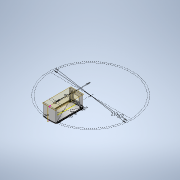
# Autodesk Inventor part: bat_mount001
Saved by Autodesk Inventor 2020 (Build 240168000, 168)
## iProperties
Created: 2024-02-10
Part Number: bat_mount001
Material: Типовые
Document SubType Name: Modeling
Designer: 4s
Density: 1 g/cm^3
Appearance: По умолчанию
Author: 4s
Autodesk Inventor part; units mm, degrees
ref_plane "YZ Plane" through (0, 0, 0) normal (1, 0, 0) x (0, 1, 0)
ref_plane "XZ Plane" through (0, 0, 0) normal (0, 1, 0) x (-1, 0, 0)
ref_plane "XY Plane" through (0, 0, 0) normal (0, 0, 1) x (1, 0, 0)
sketch "Эскиз1" plane through (0, 0, 0) normal (0, 1, 0) x (-1, 0, 0)
  circle A0 centre (0, 0) radius 101 construction
  line L0 (0, 0) -> (0, 101) construction
  line L1 (101, 0) -> (-101, 0) construction
  line L2 (16.8284, 102.0346) -> (-15, 102.0346)
  line L3 (-15, 100.0346) -> (-15, 37.0346)
  line L4 (-13, 37.0346) -> (13, 37.0346)
  line L5 (15, 37.0346) -> (15, 100.0346)
  line L6 (15, 102.0346) -> (-15, 37.0346) construction
  line L7 (-15, 102.0346) -> (15, 37.0346) construction
  arc A1 (15, 100.0346) -> (13, 102.0346) centre (13, 100.0346) ccw
  arc A2 (13, 37.0346) -> (15, 39.0346) centre (13, 39.0346) ccw
  arc A3 (-15, 39.0346) -> (-13, 37.0346) centre (-13, 39.0346) ccw
  arc A4 (-13, 102.0346) -> (-15, 100.0346) centre (-13, 100.0346) ccw
  line L8 (14, 104.0346) -> (-14, 104.0346) construction
  line L9 (-17, 101.0346) -> (-17, 38.0346)
  line L10 (-14, 35.0346) -> (14, 35.0346)
  line L11 (17, 38.0346) -> (17, 101.0346)
  line L12 (17, 104.0346) -> (-17, 35.0346) construction
  line L13 (-17, 104.0346) -> (17, 35.0346) construction
  arc A5 (14, 35.0346) -> (17, 38.0346) centre (14, 38.0346) ccw
  arc A6 (-17, 38.0346) -> (-14, 35.0346) centre (-14, 38.0346) ccw
  arc A7 (-14, 104.0346) -> (-17, 101.0346) centre (-14, 101.0346) ccw
  arc A8 (17, 101.0346) -> (14, 104.0346) centre (14, 101.0346) ccw
  arc A9 (-14.4118, 104.0063) -> (14.4118, 104.0063) centre (0, 0) ccw construction
  arc A10 (14.4118, 104.0063) -> (-14.4118, 104.0063) centre (0, 0) ccw
  line L14 (-15, 102.0346) -> (-16.8284, 102.0346)
  line L15 (-15, 37.0346) -> (-15, 35.2062)
  line L16 (15, 37.0346) -> (15, 35.2062)
  point P0 (0, 69.5346)
  dimension "d2" = 202
  dimension "d3" = 30
  dimension "d4" = 65
  dimension "d5" = 2
  dimension "d6" = 2
  dimension "d7" = 2
  dimension "d8" = 3
  dimension "d9" = 210
  constraints: 34 end point, 29 point on circle, 18 point on line, 17 tangent, 11 centre point, 6 equal radius, 5 midpoint, 4 horizontal, 4 parallel, 3 vertical, 2 coincident, 2 perpendicular, 1 other
  measures "d2" diameter of A0
  measures "d3" distance of L5.start L3.end
  measures "d4" distance of L3.end L2.end
  measures "d5" radius of A1
  measures "d6" distance between parallel lines of L3 L9
  measures "d7" distance between parallel lines of L10 L4
  measures "d8" radius of A5
  measures "d9" diameter of A9
extrude "Выдавливание3" add sketch "Эскиз1" against normal blind 2
ref_plane "РабПлоскость1" through (0, 28, 0) normal (0, 1, 0) x (1, 0, 0)
extrude "Выдавливание1" add sketch "Эскиз1" along normal up to surface (28 mm away) contours L2 L14 A7 A10 A8
ref_plane "РабПлоскость2" through (0, 7, 101.0346) normal (1, 0, 0) x (0, 0, -1)
sketch "Эскиз2" plane through (0, 7, 101.0346) normal (1, 0, 0) x (0, 0, -1)
  line L0 (-1, 0) -> (-1, 21) construction
  line L1 (-1, 21) -> (-2.9716, 21) construction
  line L2 (-2.9716, -9) -> (-2.9716, 21) construction
  line L3 (-2.9716, -9) -> (-2.9716, 21) construction
  line L4 (-2.9716, -9) -> (-2.9716, -9) construction
  line L5 (-2.9716, -9) -> (-2.9716, 21) construction
  line L6 (-2.9716, 21) -> (-2.9716, 21) construction
  line L7 (-2.9716, 21) -> (-2.9716, 21) construction
  line L8 (-1, 21) -> (-2.9716, 21) construction
  line L9 (-2.9716, 21) -> (-1, 21) construction
  line L10 (-1, -7) -> (0, -7) projected
  line L11 (0, -7) -> (63, -7) projected
  line L12 (63, -7) -> (66, -7) projected
  line L13 (66, -7) -> (63, -7) projected
  line L14 (63, -7) -> (0, -7) projected
  line L15 (0, -7) -> (-1, -7) projected
  point P0 (101.0346, -7)
extrude "Выдавливание4" add sketch "Эскиз1" along normal up to surface (28 mm away) contours L5 L16 A5 L10 A6 L15 L3 A3 L4 A2
sketch "Эскиз3" plane through (14, -2, 35.0346) normal (0, 0, -1) x (-1, 0, 0)
  line L0 (0, 0) -> (0, 30) construction
  line L1 (28, 0) -> (0, 0) construction
  line L2 (28, 0) -> (28, 30) construction
  line L3 (28, 30) -> (0, 30) construction
  line L4 (30.8284, 30) -> (-2.8284, 30) construction
  line L5 (-2.8284, 2) -> (-2.8284, 30) construction
  line L6 (30.8284, 2) -> (-2.8284, 2) construction
  line L7 (30.8284, 2) -> (30.8284, 30) construction
  line L8 (-3, 2) -> (-1, 2) construction
  line L9 (-3, 2) -> (-3, 0) construction
  line L10 (0, 0) -> (-3, 0) construction
  line L11 (0, 0) -> (0, 30) construction
  line L12 (0, 30) -> (-1, 30) construction
  line L13 (-1, 2) -> (-1, 30) construction
  line L14 (28.4118, 0) -> (28.4118, 30) construction
  line L15 (28, 0) -> (28, 30) construction
  line L16 (31, 0) -> (28, 0) construction
  line L17 (31, 2) -> (31, 0) construction
  line L18 (29, 2) -> (31, 2) construction
  line L19 (29, 2) -> (29, 30) construction
  line L20 (29, 30) -> (28, 30) construction
  line L21 (-0.4118, 0) -> (-0.4118, 30) construction
  line L22 (1, 30) -> (27, 30) construction
  line L23 (14, 30) -> (14, 2) construction
  line L24 (9, 9) -> (19, 9)
  line L25 (22, 12) -> (22, 19)
  line L26 (19, 22) -> (9, 22)
  line L27 (6, 19) -> (6, 12)
  line L28 (6, 9) -> (22, 22) construction
  line L29 (22, 9) -> (6, 22) construction
  arc A0 (9, 22) -> (6, 19) centre (9, 19) ccw
  arc A1 (22, 19) -> (19, 22) centre (19, 19) ccw
  arc A2 (19, 9) -> (22, 12) centre (19, 12) ccw
  arc A3 (6, 12) -> (9, 9) centre (9, 12) ccw
  point P0 (14, 15.5)
  dimension "d19" = 16
  dimension "d20" = 13
  dimension "d21" = 7
  dimension "d22" = 3
  constraints: 14 end point, 9 point on line, 8 point on circle, 8 tangent, 4 centre point, 3 equal radius, 3 midpoint, 2 parallel, 1 horizontal, 1 perpendicular, 1 vertical
  measures "d19" distance of L29.end L28.end
  measures "d20" distance of L28.end L29.start
  measures "d21" distance between parallel lines of L6 L24
  measures "d22" radius of A0
extrude "Выдавливание5" cut sketch "Эскиз3" against normal blind 10
sketch "Эскиз4" plane through (0, 28, 0) normal (0, 1, 0) x (1, 0, 0)
  line L0 (0, 0) -> (0, -84) construction
  line L1 (0, -84) -> (0, -89) construction
  line L2 (0, -89) -> (0, -84) construction
  line L3 (0, -84) -> (-17, -84) construction
  line L4 (-17, -84) -> (-17, -89) construction
  line L5 (-17, -89) -> (0, -89) construction
  line L6 (0, -84) -> (17, -84) construction
  line L7 (17, -89) -> (0, -89) construction
  line L8 (0, -84) -> (0, -34) construction
  dimension "d25" = 84
  dimension "d26" = 5
  dimension "d27" = 50
  constraints: 18 end point, 3 equal length, 2 point on line, 2 symmetric about line, 1 perpendicular, 1 vertical
  measures "d25" distance of L0.start L0.end
  measures "d26" distance of L0.end L1.end
  measures "d27" distance of L0.end L8.end
